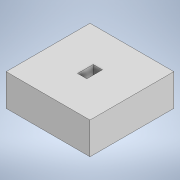
# Autodesk Inventor part: Motor_fit_check
Saved by Autodesk Inventor 2022 (Build 260153000, 153)
## iProperties
Created: 2023-02-21
Part Number: Motor_fit_check
Material: Generic
Document SubType Name: Modeling
Designer: zarek
Density: 1 g/cm^3
Appearance: Default
Author: zarek
Autodesk Inventor part; units mm, degrees
ref_plane "YZ Plane" through (0, 0, 0) normal (1, 0, 0) x (0, 1, 0)
ref_plane "XZ Plane" through (0, 0, 0) normal (0, 1, 0) x (-1, 0, 0)
ref_plane "XY Plane" through (0, 0, 0) normal (0, 0, 1) x (1, 0, 0)
sketch "Sketch1" plane through (0, 0, 0) normal (0, 1, 0) x (-1, 0, 0)
  line L0 (14.5, -14.5) -> (-14.5, -14.5)
  line L1 (-14.5, -14.5) -> (-14.5, 14.5)
  line L2 (-14.5, 14.5) -> (14.5, 14.5)
  line L3 (14.5, 14.5) -> (14.5, -14.5)
  dimension "d11" = 29
  dimension "d14" = 29
  constraints: 8 end point, 2 parallel, 1 horizontal, 1 perpendicular
  measures "d11" distance between parallel lines of L1 L3
  measures "d14" distance between parallel lines of L2 L0
extrude "Extrusion1" add sketch "Sketch1" along normal blind 11
sketch "Sketch5" plane through (0, 11, 0) normal (0, 1, 0) x (1, 0, 0)
  line L0 (-1.6, 2.7) -> (1.6, 2.7)
  line L1 (1.6, 2.7) -> (1.6, -2.7)
  line L2 (1.6, -2.7) -> (-1.6, -2.7)
  line L3 (-1.6, -2.7) -> (-1.6, 2.7)
  point P0 (0, 0)
  dimension "d31" = 2.7
  dimension "d32" = 2.7
  dimension "d33" = 3.2
  dimension "d34" = 1.6
  constraints: 8 end point, 2 parallel, 1 horizontal, 1 perpendicular
  measures "d31" distance from line of L0 point (0, 0)
  measures "d32" distance from line of L2 point (0, 0)
  measures "d33" distance between parallel lines of L1 L3
  measures "d34" distance from line of L1 point (0, 0)
extrude "Extrusion4" cut sketch "Sketch5" against normal blind 6
equation "\"d14\" = d11"
equation "\"d34\" = 0.5 * d33"
body "Solid1"
